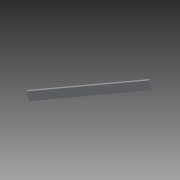
# Autodesk Inventor part: nd-m
Saved by Autodesk Inventor 2015 (Build 190159000, 159)
## iProperties
Created: 2014-07-02
Part Number: nd-m
Material: Generic
Document SubType Name: Modeling
Designer: peter
Density: 1 g/cm^3
Appearance: Default
Author: peter
Autodesk Inventor part; units mm, degrees
ref_plane "YZ Plane" through (0, 0, 0) normal (1, 0, 0) x (0, 1, 0)
ref_plane "XZ Plane" through (0, 0, 0) normal (0, 1, 0) x (-1, 0, 0)
ref_plane "XY Plane" through (0, 0, 0) normal (0, 0, 1) x (1, 0, 0)
sketch "Sketch1" plane through (0, 0, 0) normal (0, 0, 1) x (1, 0, 0)
  line L0 (25.3573, 0.0854) -> (-0.0427, 44.0795)
  line L1 (-0.0427, 44.0795) -> (834.3444, 525.8131)
  line L2 (834.3444, 525.8131) -> (859.7444, 481.819)
  line L3 (859.7444, 481.819) -> (25.3573, 0.0854)
  point P0 (0, 0)
  constraints: 8 end point
extrude "Extrusion1" add sketch "Sketch1" along normal blind 19.05
body "Solid1"
